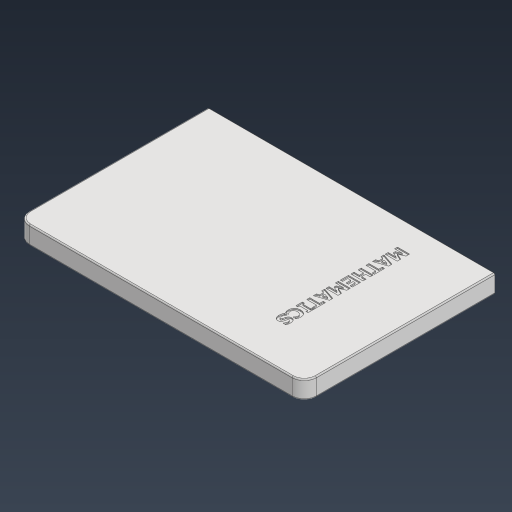
# Autodesk Inventor part: kindle
Saved by Autodesk Inventor 2023 (Build 270158000, 158)
## iProperties
Created: 2026-01-24
Part Number: kindle
Material: Generic
Document SubType Name: Modeling
Designer: szymo
Density: 1 g/cm^3
Appearance: Default
Author: szymo
Autodesk Inventor part; units mm, degrees
ref_plane "YZ Plane" through (0, 0, 0) normal (1, 0, 0) x (0, 1, 0)
ref_plane "XZ Plane" through (0, 0, 0) normal (0, 1, 0) x (-1, 0, 0)
ref_plane "XY Plane" through (0, 0, 0) normal (0, 0, 1) x (1, 0, 0)
sketch "Sketch1" plane through (0, 0, 0) normal (0, 1, 0) x (-1, 0, 0)
  line L0 (0, 0) -> (-238.048, 0)
  line L1 (-238.048, 0) -> (-238.048, 158.0036)
  line L2 (-238.048, 158.0036) -> (0, 158.0036)
  line L3 (0, 158.0036) -> (0, 0)
  constraints: 8 end point, 2 parallel, 1 horizontal, 1 perpendicular
extrude "Extrusion1" add sketch "Sketch1" along normal blind 15
sketch "Sketch2" plane through (0, 15, 0) normal (0, 1, 0) x (1, 0, 0)
  line L0 (188.9981, -20.4189) -> (188.9981, -48.4017) construction
  line L1 (188.9981, -48.4017) -> (199.0594, -48.4017) construction
  line L2 (199.0594, -48.4017) -> (199.0594, -20.4189) construction
  line L3 (199.0594, -20.4189) -> (188.9981, -20.4189) construction
  line L4 (178.8036, -31.6669) -> (178.8036, -29.1709)
  line L5 (178.8036, -29.1709) -> (185.4324, -29.1709)
  line L6 (185.4324, -29.1709) -> (181.1537, -27.3557)
  line L7 (181.1537, -27.3557) -> (181.1537, -25.6377)
  line L8 (181.1537, -25.6377) -> (185.4324, -23.8225)
  line L9 (185.4324, -23.8225) -> (178.8036, -23.8225)
  line L10 (178.8036, -23.8225) -> (178.8036, -21.4562)
  line L11 (178.8036, -21.4562) -> (188.8036, -21.4562)
  line L12 (188.8036, -21.4562) -> (188.8036, -24.3492)
  line L13 (188.8036, -24.3492) -> (183.8684, -26.5696)
  line L14 (183.8684, -26.5696) -> (188.8036, -28.7738)
  line L15 (188.8036, -28.7738) -> (188.8036, -31.6669)
  line L16 (188.8036, -31.6669) -> (178.8036, -31.6669)
  line L17 (178.8036, -32.6636) -> (188.8036, -36.0429)
  line L18 (188.8036, -36.0429) -> (188.8036, -38.7819)
  line L19 (188.8036, -38.7819) -> (178.8036, -42.1612)
  line L20 (178.8036, -42.1612) -> (178.8036, -39.5761)
  line L21 (178.8036, -39.5761) -> (180.8457, -38.9521)
  line L22 (180.8457, -38.9521) -> (180.8457, -35.8079)
  line L23 (180.8457, -35.8079) -> (178.8036, -35.1758)
  line L24 (178.8036, -35.1758) -> (178.8036, -32.6636)
  line L25 (182.6609, -38.4011) -> (185.9673, -37.38)
  line L26 (185.9673, -37.38) -> (182.6609, -36.3508)
  line L27 (182.6609, -36.3508) -> (182.6609, -38.4011)
  line L28 (178.8036, -45.0785) -> (186.8992, -45.0785)
  line L29 (186.8992, -45.0785) -> (186.8992, -42.1207)
  line L30 (186.8992, -42.1207) -> (188.8036, -42.1207)
  line L31 (188.8036, -42.1207) -> (188.8036, -50.5485)
  line L32 (188.8036, -50.5485) -> (186.8992, -50.5485)
  line L33 (186.8992, -50.5485) -> (186.8992, -47.5907)
  line L34 (186.8992, -47.5907) -> (178.8036, -47.5907)
  line L35 (178.8036, -47.5907) -> (178.8036, -45.0785)
  line L36 (178.8036, -60.0137) -> (178.8036, -57.5015)
  line L37 (178.8036, -57.5015) -> (183.2363, -57.5015)
  line L38 (183.2363, -57.5015) -> (183.2363, -54.0899)
  line L39 (183.2363, -54.0899) -> (178.8036, -54.0899)
  line L40 (178.8036, -54.0899) -> (178.8036, -51.5777)
  line L41 (178.8036, -51.5777) -> (188.8036, -51.5777)
  line L42 (188.8036, -51.5777) -> (188.8036, -54.0899)
  line L43 (188.8036, -54.0899) -> (185.1407, -54.0899)
  line L44 (185.1407, -54.0899) -> (185.1407, -57.5015)
  line L45 (185.1407, -57.5015) -> (188.8036, -57.5015)
  line L46 (188.8036, -57.5015) -> (188.8036, -60.0137)
  line L47 (188.8036, -60.0137) -> (178.8036, -60.0137)
  line L48 (178.8036, -62.0883) -> (188.8036, -62.0883)
  line L49 (188.8036, -62.0883) -> (188.8036, -68.8468)
  line L50 (188.8036, -68.8468) -> (186.8992, -68.8468)
  line L51 (186.8992, -68.8468) -> (186.8992, -64.5842)
  line L52 (186.8992, -64.5842) -> (185.1407, -64.5842)
  line L53 (185.1407, -64.5842) -> (185.1407, -68.5145)
  line L54 (185.1407, -68.5145) -> (183.2363, -68.5145)
  line L55 (183.2363, -68.5145) -> (183.2363, -64.5842)
  line L56 (183.2363, -64.5842) -> (180.7079, -64.5842)
  line L57 (180.7079, -64.5842) -> (180.7079, -68.8468)
  line L58 (180.7079, -68.8468) -> (178.8036, -68.8468)
  line L59 (178.8036, -68.8468) -> (178.8036, -62.0883)
  line L60 (178.8036, -80.7592) -> (178.8036, -78.2633)
  line L61 (178.8036, -78.2633) -> (185.4324, -78.2633)
  line L62 (185.4324, -78.2633) -> (181.1537, -76.4481)
  line L63 (181.1537, -76.4481) -> (181.1537, -74.7301)
  line L64 (181.1537, -74.7301) -> (185.4324, -72.9148)
  line L65 (185.4324, -72.9148) -> (178.8036, -72.9148)
  line L66 (178.8036, -72.9148) -> (178.8036, -70.5485)
  line L67 (178.8036, -70.5485) -> (188.8036, -70.5485)
  line L68 (188.8036, -70.5485) -> (188.8036, -73.4416)
  line L69 (188.8036, -73.4416) -> (183.8684, -75.662)
  line L70 (183.8684, -75.662) -> (188.8036, -77.8662)
  line L71 (188.8036, -77.8662) -> (188.8036, -80.7592)
  line L72 (188.8036, -80.7592) -> (178.8036, -80.7592)
  line L73 (178.8036, -81.756) -> (188.8036, -85.1353)
  line L74 (188.8036, -85.1353) -> (188.8036, -87.8743)
  line L75 (188.8036, -87.8743) -> (178.8036, -91.2536)
  line L76 (178.8036, -91.2536) -> (178.8036, -88.6685)
  line L77 (178.8036, -88.6685) -> (180.8457, -88.0445)
  line L78 (180.8457, -88.0445) -> (180.8457, -84.9003)
  line L79 (180.8457, -84.9003) -> (178.8036, -84.2682)
  line L80 (178.8036, -84.2682) -> (178.8036, -81.756)
  line L81 (182.6609, -87.4934) -> (185.9673, -86.4724)
  line L82 (185.9673, -86.4724) -> (182.6609, -85.4432)
  line L83 (182.6609, -85.4432) -> (182.6609, -87.4934)
  line L84 (178.8036, -94.1709) -> (186.8992, -94.1709)
  line L85 (186.8992, -94.1709) -> (186.8992, -91.2131)
  line L86 (186.8992, -91.2131) -> (188.8036, -91.2131)
  line L87 (188.8036, -91.2131) -> (188.8036, -99.6409)
  line L88 (188.8036, -99.6409) -> (186.8992, -99.6409)
  line L89 (186.8992, -99.6409) -> (186.8992, -96.6831)
  line L90 (186.8992, -96.6831) -> (178.8036, -96.6831)
  line L91 (178.8036, -96.6831) -> (178.8036, -94.1709)
  line L92 (178.8036, -105.6458) -> (178.8036, -100.2649)
  line L93 (178.8036, -100.2649) -> (180.5459, -100.2649)
  line L94 (180.5459, -100.2649) -> (180.5459, -101.6993)
  line L95 (180.5459, -101.6993) -> (187.0613, -101.6993)
  line L96 (187.0613, -101.6993) -> (187.0613, -100.2649)
  line L97 (187.0613, -100.2649) -> (188.8036, -100.2649)
  line L98 (188.8036, -100.2649) -> (188.8036, -105.6458)
  line L99 (188.8036, -105.6458) -> (187.0613, -105.6458)
  line L100 (187.0613, -105.6458) -> (187.0613, -104.2114)
  line L101 (187.0613, -104.2114) -> (180.5459, -104.2114)
  line L102 (180.5459, -104.2114) -> (180.5459, -105.6458)
  line L103 (180.5459, -105.6458) -> (178.8036, -105.6458)
  spline S0 degree 2 poles (178.6091, -111.6263) (178.6091, -109.3735) (181.3319, -106.7317) (183.7955, -106.7317) knots 0 0 0 1 2 2 2
  spline S1 degree 2 poles (183.7955, -106.7317) (186.1699, -106.7317) (188.9981, -109.3816) (188.9981, -111.6344) knots 0 0 0 1 2 2 2
  spline S2 degree 2 poles (188.9981, -111.6344) (188.9981, -112.226) (188.8603, -113.1823) (188.7468, -113.6199) knots 0 0 0 1 2 2 2
  spline S3 degree 2 poles (188.7468, -113.6199) (188.6415, -113.9602) (188.293, -114.7625) (188.1634, -115.0137) knots 0 0 0 1 2 2 2
  line L104 (188.1634, -115.0137) -> (185.7809, -115.0137)
  line L105 (185.7809, -115.0137) -> (185.7809, -114.7625)
  spline S4 degree 2 poles (185.7809, -114.7625) (185.943, -114.5761) (186.3968, -114.025) (186.6075, -113.6766) knots 0 0 0 1 2 2 2
  spline S5 degree 2 poles (186.6075, -113.6766) (186.8263, -113.3281) (187.1261, -112.4934) (187.1261, -112.0315) knots 0 0 0 1 2 2 2
  spline S6 degree 2 poles (187.1261, -112.0315) (187.1261, -111.4886) (186.7857, -110.5891) (186.3562, -110.1758) knots 0 0 0 1 2 2 2
  spline S7 degree 2 poles (186.3562, -110.1758) (185.9754, -109.803) (184.6707, -109.3249) (183.7874, -109.3249) knots 0 0 0 1 2 2 2
  spline S8 degree 2 poles (183.7874, -109.3249) (182.8554, -109.3249) (181.5831, -109.8192) (181.1942, -110.2244) knots 0 0 0 1 2 2 2
  spline S9 degree 2 poles (181.1942, -110.2244) (180.8133, -110.6134) (180.481, -111.5696) (180.481, -112.0477) knots 0 0 0 1 2 2 2
  spline S10 degree 2 poles (180.481, -112.0477) (180.481, -112.5421) (180.8133, -113.4416) (181.0159, -113.7495) knots 0 0 0 1 2 2 2
  spline S11 degree 2 poles (181.0159, -113.7495) (181.2185, -114.0899) (181.648, -114.6004) (181.8182, -114.7868) knots 0 0 0 1 2 2 2
  line L106 (181.8182, -114.7868) -> (181.8182, -115.0137)
  line L107 (181.8182, -115.0137) -> (179.4681, -115.0137)
  spline S12 degree 2 poles (179.4681, -115.0137) (179.3384, -114.7382) (179.0143, -114.0169) (178.9008, -113.628) knots 0 0 0 1 2 2 2
  spline S13 degree 2 poles (178.9008, -113.628) (178.7549, -113.1579) (178.6091, -112.3395) (178.6091, -111.6263) knots 0 0 0 1 2 2 2
  spline S14 degree 2 poles (178.6253, -119.5842) (178.6253, -118.4335) (179.071, -116.6993) (179.3951, -115.9537) knots 0 0 0 1 2 2 2
  line L108 (179.3951, -115.9537) -> (181.7776, -115.9537)
  line L109 (181.7776, -115.9537) -> (181.7776, -116.1806)
  spline S15 degree 2 poles (181.7776, -116.1806) (181.1374, -116.9343) (180.4486, -118.7414) (180.4486, -119.5923) knots 0 0 0 1 2 2 2
  spline S16 degree 2 poles (180.4486, -119.5923) (180.4486, -119.8111) (180.5459, -120.5161) (180.6431, -120.7268) knots 0 0 0 1 2 2 2
  spline S17 degree 2 poles (180.6431, -120.7268) (180.7566, -120.9861) (181.1699, -121.3508) (181.5021, -121.3508) knots 0 0 0 1 2 2 2
  spline S18 degree 2 poles (181.5021, -121.3508) (181.883, -121.3508) (182.353, -120.7592) (182.4584, -120.3541) knots 0 0 0 1 2 2 2
  spline S19 degree 2 poles (182.4584, -120.3541) (182.5961, -119.8435) (182.8311, -118.6847) (183.0094, -118.1742) knots 0 0 0 1 2 2 2
  spline S20 degree 2 poles (183.0094, -118.1742) (183.4146, -117.0153) (184.8003, -116.0105) (185.8376, -116.0105) knots 0 0 0 1 2 2 2
  spline S21 degree 2 poles (185.8376, -116.0105) (187.2396, -116.0105) (188.9819, -118.3849) (188.9819, -120.1677) knots 0 0 0 1 2 2 2
  spline S22 degree 2 poles (188.9819, -120.1677) (188.9819, -121.0591) (188.6172, -122.8257) (188.3092, -123.5226) knots 0 0 0 1 2 2 2
  line L110 (188.3092, -123.5226) -> (186.024, -123.5226)
  line L111 (186.024, -123.5226) -> (186.024, -123.3038)
  spline S23 degree 2 poles (186.024, -123.3038) (186.5021, -122.7447) (187.1585, -121.1401) (187.1585, -120.2973) knots 0 0 0 1 2 2 2
  spline S24 degree 2 poles (187.1585, -120.2973) (187.1585, -119.9651) (187.0613, -119.4464) (186.9316, -119.1547) knots 0 0 0 1 2 2 2
  spline S25 degree 2 poles (186.9316, -119.1547) (186.8263, -118.9197) (186.4049, -118.5793) (186.1455, -118.5793) knots 0 0 0 1 2 2 2
  spline S26 degree 2 poles (186.1455, -118.5793) (185.7566, -118.5793) (185.3109, -119.1223) (185.1326, -119.9003) knots 0 0 0 1 2 2 2
  spline S27 degree 2 poles (185.1326, -119.9003) (185.0191, -120.4027) (184.8003, -121.3346) (184.6139, -121.8695) knots 0 0 0 1 2 2 2
  spline S28 degree 2 poles (184.6139, -121.8695) (184.2331, -122.9067) (182.9689, -123.9197) (181.9316, -123.9197) knots 0 0 0 1 2 2 2
  spline S29 degree 2 poles (181.9316, -123.9197) (180.4405, -123.9197) (178.6253, -121.5777) (178.6253, -119.5842) knots 0 0 0 1 2 2 2
  point P0 (0, 0)
  constraints: 2 other
extrude "Extrusion2" cut sketch "Sketch2" against normal blind 1
fillet "Fillet1" radius 10 2 edges at (0, 7.5, 158.0036) (238.048, 7.5, 158.0036)
fillet "Fillet2" radius 1 10 edges at (235.1191, 15, 155.0746) (119.024, 15, 158.0036) (2.9289, 15, 155.0746) (0, 15, 74.0018) (238.048, 15, 74.0018) (235.1191, 0, 155.0746) (238.048, 0, 74.0018) (2.9289, 0, 155.0746) (0, 0, 74.0018) (119.024, 0, 158.0036)
sketch "Sketch3" plane through (237.048, 0, 0) normal (0, 0, -1) x (-1, 0, 0)
  line L0 (10.3875, 9.9835) -> (56.291, 9.9835) construction
  line L1 (56.291, 9.9835) -> (56.291, 4.8052) construction
  line L2 (56.291, 4.8052) -> (10.3875, 4.8052) construction
  line L3 (10.3875, 4.8052) -> (10.3875, 9.9835) construction
  line L4 (16.0115, 4.8863) -> (14.7635, 4.8863)
  line L5 (14.7635, 4.8863) -> (14.7635, 8.2007)
  line L6 (14.7635, 8.2007) -> (13.8559, 6.0613)
  line L7 (13.8559, 6.0613) -> (12.9969, 6.0613)
  line L8 (12.9969, 6.0613) -> (12.0893, 8.2007)
  line L9 (12.0893, 8.2007) -> (12.0893, 4.8863)
  line L10 (12.0893, 4.8863) -> (10.9061, 4.8863)
  line L11 (10.9061, 4.8863) -> (10.9061, 9.8863)
  line L12 (10.9061, 9.8863) -> (12.3526, 9.8863)
  line L13 (12.3526, 9.8863) -> (13.4628, 7.4187)
  line L14 (13.4628, 7.4187) -> (14.565, 9.8863)
  line L15 (14.565, 9.8863) -> (16.0115, 9.8863)
  line L16 (16.0115, 9.8863) -> (16.0115, 4.8863)
  line L17 (16.5099, 4.8863) -> (18.1995, 9.8863)
  line L18 (18.1995, 9.8863) -> (19.569, 9.8863)
  line L19 (19.569, 9.8863) -> (21.2586, 4.8863)
  line L20 (21.2586, 4.8863) -> (19.9661, 4.8863)
  line L21 (19.9661, 4.8863) -> (19.6541, 5.9073)
  line L22 (19.6541, 5.9073) -> (18.082, 5.9073)
  line L23 (18.082, 5.9073) -> (17.7659, 4.8863)
  line L24 (17.7659, 4.8863) -> (16.5099, 4.8863)
  line L25 (19.3786, 6.8149) -> (18.868, 8.4681)
  line L26 (18.868, 8.4681) -> (18.3534, 6.8149)
  line L27 (18.3534, 6.8149) -> (19.3786, 6.8149)
  line L28 (22.7173, 4.8863) -> (22.7173, 8.9341)
  line L29 (22.7173, 8.9341) -> (21.2384, 8.9341)
  line L30 (21.2384, 8.9341) -> (21.2384, 9.8863)
  line L31 (21.2384, 9.8863) -> (25.4523, 9.8863)
  line L32 (25.4523, 9.8863) -> (25.4523, 8.9341)
  line L33 (25.4523, 8.9341) -> (23.9734, 8.9341)
  line L34 (23.9734, 8.9341) -> (23.9734, 4.8863)
  line L35 (23.9734, 4.8863) -> (22.7173, 4.8863)
  line L36 (30.1849, 4.8863) -> (28.9288, 4.8863)
  line L37 (28.9288, 4.8863) -> (28.9288, 7.1026)
  line L38 (28.9288, 7.1026) -> (27.223, 7.1026)
  line L39 (27.223, 7.1026) -> (27.223, 4.8863)
  line L40 (27.223, 4.8863) -> (25.9669, 4.8863)
  line L41 (25.9669, 4.8863) -> (25.9669, 9.8863)
  line L42 (25.9669, 9.8863) -> (27.223, 9.8863)
  line L43 (27.223, 9.8863) -> (27.223, 8.0548)
  line L44 (27.223, 8.0548) -> (28.9288, 8.0548)
  line L45 (28.9288, 8.0548) -> (28.9288, 9.8863)
  line L46 (28.9288, 9.8863) -> (30.1849, 9.8863)
  line L47 (30.1849, 9.8863) -> (30.1849, 4.8863)
  line L48 (31.2222, 4.8863) -> (31.2222, 9.8863)
  line L49 (31.2222, 9.8863) -> (34.6014, 9.8863)
  line L50 (34.6014, 9.8863) -> (34.6014, 8.9341)
  line L51 (34.6014, 8.9341) -> (32.4701, 8.9341)
  line L52 (32.4701, 8.9341) -> (32.4701, 8.0548)
  line L53 (32.4701, 8.0548) -> (34.4353, 8.0548)
  line L54 (34.4353, 8.0548) -> (34.4353, 7.1026)
  line L55 (34.4353, 7.1026) -> (32.4701, 7.1026)
  line L56 (32.4701, 7.1026) -> (32.4701, 5.8384)
  line L57 (32.4701, 5.8384) -> (34.6014, 5.8384)
  line L58 (34.6014, 5.8384) -> (34.6014, 4.8863)
  line L59 (34.6014, 4.8863) -> (31.2222, 4.8863)
  line L60 (40.5577, 4.8863) -> (39.3097, 4.8863)
  line L61 (39.3097, 4.8863) -> (39.3097, 8.2007)
  line L62 (39.3097, 8.2007) -> (38.4021, 6.0613)
  line L63 (38.4021, 6.0613) -> (37.5431, 6.0613)
  line L64 (37.5431, 6.0613) -> (36.6355, 8.2007)
  line L65 (36.6355, 8.2007) -> (36.6355, 4.8863)
  line L66 (36.6355, 4.8863) -> (35.4523, 4.8863)
  line L67 (35.4523, 4.8863) -> (35.4523, 9.8863)
  line L68 (35.4523, 9.8863) -> (36.8988, 9.8863)
  line L69 (36.8988, 9.8863) -> (38.009, 7.4187)
  line L70 (38.009, 7.4187) -> (39.1111, 9.8863)
  line L71 (39.1111, 9.8863) -> (40.5577, 9.8863)
  line L72 (40.5577, 9.8863) -> (40.5577, 4.8863)
  line L73 (41.056, 4.8863) -> (42.7457, 9.8863)
  line L74 (42.7457, 9.8863) -> (44.1152, 9.8863)
  line L75 (44.1152, 9.8863) -> (45.8048, 4.8863)
  line L76 (45.8048, 4.8863) -> (44.5123, 4.8863)
  line L77 (44.5123, 4.8863) -> (44.2003, 5.9073)
  line L78 (44.2003, 5.9073) -> (42.6282, 5.9073)
  line L79 (42.6282, 5.9073) -> (42.3121, 4.8863)
  line L80 (42.3121, 4.8863) -> (41.056, 4.8863)
  line L81 (43.9248, 6.8149) -> (43.4142, 8.4681)
  line L82 (43.4142, 8.4681) -> (42.8996, 6.8149)
  line L83 (42.8996, 6.8149) -> (43.9248, 6.8149)
  line L84 (47.2635, 4.8863) -> (47.2635, 8.9341)
  line L85 (47.2635, 8.9341) -> (45.7846, 8.9341)
  line L86 (45.7846, 8.9341) -> (45.7846, 9.8863)
  line L87 (45.7846, 9.8863) -> (49.9985, 9.8863)
  line L88 (49.9985, 9.8863) -> (49.9985, 8.9341)
  line L89 (49.9985, 8.9341) -> (48.5196, 8.9341)
  line L90 (48.5196, 8.9341) -> (48.5196, 4.8863)
  line L91 (48.5196, 4.8863) -> (47.2635, 4.8863)
  line L92 (53.0009, 4.8863) -> (50.3105, 4.8863)
  line L93 (50.3105, 4.8863) -> (50.3105, 5.7574)
  line L94 (50.3105, 5.7574) -> (51.0277, 5.7574)
  line L95 (51.0277, 5.7574) -> (51.0277, 9.0151)
  line L96 (51.0277, 9.0151) -> (50.3105, 9.0151)
  line L97 (50.3105, 9.0151) -> (50.3105, 9.8863)
  line L98 (50.3105, 9.8863) -> (53.0009, 9.8863)
  line L99 (53.0009, 9.8863) -> (53.0009, 9.0151)
  line L100 (53.0009, 9.0151) -> (52.2838, 9.0151)
  line L101 (52.2838, 9.0151) -> (52.2838, 5.7574)
  line L102 (52.2838, 5.7574) -> (53.0009, 5.7574)
  line L103 (53.0009, 5.7574) -> (53.0009, 4.8863)
  spline S0 degree 2 poles (55.9912, 4.789) (54.8648, 4.789) (53.5439, 6.1504) (53.5439, 7.3822) knots 0 0 0 1 2 2 2
  spline S1 degree 2 poles (53.5439, 7.3822) (53.5439, 8.5694) (54.8688, 9.9835) (55.9953, 9.9835) knots 0 0 0 1 2 2 2
  spline S2 degree 2 poles (55.9953, 9.9835) (56.2911, 9.9835) (56.7692, 9.9146) (56.988, 9.8579) knots 0 0 0 1 2 2 2
  spline S3 degree 2 poles (56.988, 9.8579) (57.1581, 9.8052) (57.5593, 9.631) (57.6849, 9.5662) knots 0 0 0 1 2 2 2
  line L104 (57.6849, 9.5662) -> (57.6849, 8.3749)
  line L105 (57.6849, 8.3749) -> (57.5593, 8.3749)
  spline S4 degree 2 poles (57.5593, 8.3749) (57.4661, 8.456) (57.1906, 8.6829) (57.0163, 8.7882) knots 0 0 0 1 2 2 2
  spline S5 degree 2 poles (57.0163, 8.7882) (56.8421, 8.8976) (56.4248, 9.0475) (56.1938, 9.0475) knots 0 0 0 1 2 2 2
  spline S6 degree 2 poles (56.1938, 9.0475) (55.9223, 9.0475) (55.4726, 8.8773) (55.2659, 8.6626) knots 0 0 0 1 2 2 2
  spline S7 degree 2 poles (55.2659, 8.6626) (55.0795, 8.4722) (54.8405, 7.8198) (54.8405, 7.3782) knots 0 0 0 1 2 2 2
  spline S8 degree 2 poles (54.8405, 7.3782) (54.8405, 6.9122) (55.0876, 6.276) (55.2902, 6.0816) knots 0 0 0 1 2 2 2
  spline S9 degree 2 poles (55.2902, 6.0816) (55.4847, 5.8911) (55.9628, 5.725) (56.2019, 5.725) knots 0 0 0 1 2 2 2
  spline S10 degree 2 poles (56.2019, 5.725) (56.4491, 5.725) (56.8988, 5.8911) (57.0528, 5.9924) knots 0 0 0 1 2 2 2
  spline S11 degree 2 poles (57.0528, 5.9924) (57.223, 6.0937) (57.4782, 6.3085) (57.5714, 6.3936) knots 0 0 0 1 2 2 2
  line L106 (57.5714, 6.3936) -> (57.6849, 6.3936)
  line L107 (57.6849, 6.3936) -> (57.6849, 5.2185)
  spline S12 degree 2 poles (57.6849, 5.2185) (57.5471, 5.1537) (57.1865, 4.9916) (56.992, 4.9349) knots 0 0 0 1 2 2 2
  spline S13 degree 2 poles (56.992, 4.9349) (56.757, 4.8619) (56.3478, 4.789) (55.9912, 4.789) knots 0 0 0 1 2 2 2
  spline S14 degree 2 poles (59.9701, 4.7971) (59.3948, 4.7971) (58.5277, 5.02) (58.1549, 5.182) knots 0 0 0 1 2 2 2
  line L108 (58.1549, 5.182) -> (58.1549, 6.3733)
  line L109 (58.1549, 6.3733) -> (58.2684, 6.3733)
  spline S15 degree 2 poles (58.2684, 6.3733) (58.6452, 6.0532) (59.5487, 5.7088) (59.9742, 5.7088) knots 0 0 0 1 2 2 2
  spline S16 degree 2 poles (59.9742, 5.7088) (60.0836, 5.7088) (60.4361, 5.7574) (60.5415, 5.806) knots 0 0 0 1 2 2 2
  spline S17 degree 2 poles (60.5415, 5.806) (60.6711, 5.8628) (60.8534, 6.0694) (60.8534, 6.2355) knots 0 0 0 1 2 2 2
  spline S18 degree 2 poles (60.8534, 6.2355) (60.8534, 6.426) (60.5577, 6.661) (60.3551, 6.7136) knots 0 0 0 1 2 2 2
  spline S19 degree 2 poles (60.3551, 6.7136) (60.0998, 6.7825) (59.5204, 6.9) (59.2651, 6.9892) knots 0 0 0 1 2 2 2
  spline S20 degree 2 poles (59.2651, 6.9892) (58.6857, 7.1918) (58.1833, 7.8846) (58.1833, 8.4033) knots 0 0 0 1 2 2 2
  spline S21 degree 2 poles (58.1833, 8.4033) (58.1833, 9.1042) (59.3705, 9.9754) (60.2619, 9.9754) knots 0 0 0 1 2 2 2
  spline S22 degree 2 poles (60.2619, 9.9754) (60.7076, 9.9754) (61.5909, 9.7931) (61.9393, 9.6391) knots 0 0 0 1 2 2 2
  line L110 (61.9393, 9.6391) -> (61.9393, 8.4965)
  line L111 (61.9393, 8.4965) -> (61.8299, 8.4965)
  spline S23 degree 2 poles (61.8299, 8.4965) (61.5504, 8.7355) (60.7481, 9.0637) (60.3267, 9.0637) knots 0 0 0 1 2 2 2
  spline S24 degree 2 poles (60.3267, 9.0637) (60.1606, 9.0637) (59.9013, 9.0151) (59.7554, 8.9503) knots 0 0 0 1 2 2 2
  spline S25 degree 2 poles (59.7554, 8.9503) (59.6379, 8.8976) (59.4677, 8.6869) (59.4677, 8.5572) knots 0 0 0 1 2 2 2
  spline S26 degree 2 poles (59.4677, 8.5572) (59.4677, 8.3628) (59.7392, 8.1399) (60.1282, 8.0508) knots 0 0 0 1 2 2 2
  spline S27 degree 2 poles (60.1282, 8.0508) (60.3794, 7.994) (60.8453, 7.8846) (61.1128, 7.7914) knots 0 0 0 1 2 2 2
  spline S28 degree 2 poles (61.1128, 7.7914) (61.6314, 7.601) (62.1379, 6.9689) (62.1379, 6.4503) knots 0 0 0 1 2 2 2
  spline S29 degree 2 poles (62.1379, 6.4503) (62.1379, 5.7047) (60.9669, 4.7971) (59.9701, 4.7971) knots 0 0 0 1 2 2 2
  point P0 (237.048, 0)
  constraints: 2 other
extrude "Extrusion3" cut sketch "Sketch3" against normal blind 1
body "Solid1"
